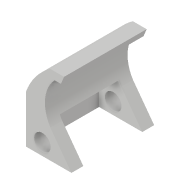
# Autodesk Inventor part: Part8
Saved by Autodesk Inventor 2017 (Build 210142000, 142)
## iProperties
Created: 2017-05-11
Part Number: Part8
Material: Generic
Document SubType Name: Modeling
Designer: zallen
Density: 1 g/cm^3
Appearance: Default
Author: zallen
Autodesk Inventor part; units mm, degrees
ref_plane "YZ Plane" through (0, 0, 0) normal (1, 0, 0) x (0, 1, 0)
ref_plane "XZ Plane" through (0, 0, 0) normal (0, 1, 0) x (-1, 0, 0)
sketch "Sketch1" plane through (0, 0, 0) normal (0, 0, 1) x (1, 0, 0)
  line L0 (0, 0) -> (0, 20)
  arc A0 (10.3297, 33.6293) -> (0, 20) centre (26.5688, 10.5925) ccw
  line L1 (10.3297, 33.6293) -> (13.2894, 33.6293)
  arc A1 (12.1727, 30.4088) -> (10.3814, 12.1465) centre (23.0461, 20.1232) ccw
  line L2 (10.3814, 12.1465) -> (19.3334, 0)
  line L3 (19.3334, 0) -> (0, 0)
  line L4 (12.1727, 30.4088) -> (14.8574, 30.4088)
  line L5 (14.8574, 30.4088) -> (16.1699, 33.6293)
  line L6 (16.1699, 33.6293) -> (13.2894, 33.6293)
  circle A2 centre (7, 5) radius 3.5
  dimension "d0" = 20
  dimension "d1" = 7
  dimension "d2" = 14.9674
  dimension "d3" = 28.1852
  dimension "d4" = 67.827
  dimension "d5" = 10.2856
  dimension "d6" = 7
  dimension "d7" = 5
  dimension "d8" = 53.61
  dimension "d9" = 3.2206
  constraints: 14 end point, 4 point on circle, 3 centre point, 3 horizontal, 1 collinear, 1 vertical
  measures "d0" distance of L0.start L0.end
  measures "d1" diameter of A2
  measures "d2" radius of A1
  measures "d3" radius of A0
  measures "d4" angle of L5 L6
  measures "d5" distance from line of A1.centre L4
  measures "d6" distance from line of L0 A2.centre
  measures "d7" distance from line of L3 A2.centre
  measures "d8" angle of L3 L2
  measures "d9" distance between parallel lines of L1 L4
extrude "Extrusion1" add sketch "Sketch1" along normal blind 35
ref_plane "Work Plane1" through (0, 0, 17.5) normal (0, 0, -1) x (-1, 0, 0)
sketch "Sketch2" plane through (0, 0, 17.5) normal (0, 0, -1) x (-1, 0, 0)
  line L0 (-1, 0) -> (-21, 0)
  line L1 (-21, 0) -> (-21, 14)
  line L2 (-21, 14) -> (-1, 14)
  line L3 (-1, 14) -> (-1, 0)
  line L4 (0, 0) -> (-25.0349, 0) construction
  dimension "d12" = 20
  dimension "d13" = 14
  dimension "d15" = 1
  constraints: 10 end point, 2 horizontal, 2 parallel, 1 perpendicular, 1 point on line
  measures "d12" distance of L1.end L2.end
  measures "d13" distance of L0.end L1.end
  measures "d15" distance of L4.start L0.start
extrude "Extrusion2" cut sketch "Sketch2" along normal mid plane 25
body "Solid1"
